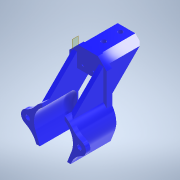
# Autodesk Inventor part: Marco Servo
Saved by Autodesk Inventor 2020.3 (Build 243373000, 373)
## iProperties
Created: 2021-02-18
Part Number: Marco Servo
Material: PET Plastic
Document SubType Name: Modeling
Designer: juanp
Density: 1.541 g/cm^3
Appearance: Polycarbonate - Clear
Author: juanp
Autodesk Inventor part; units mm, degrees
ref_plane "YZ Plane" through (0, 0, 0) normal (1, 0, 0) x (0, 1, 0)
ref_plane "XZ Plane" through (0, 0, 0) normal (0, 1, 0) x (-1, 0, 0)
ref_plane "XY Plane" through (0, 0, 0) normal (0, 0, 1) x (1, 0, 0)
sketch "Sketch1" plane through (0, 0, 0) normal (0, 0, 1) x (1, 0, 0)
  line L0 (0, 0) -> (20, 0)
  line L1 (20, 0) -> (20, 40.2)
  line L2 (20, 40.2) -> (0, 40.2)
  line L3 (0, 40.2) -> (0, 0)
  line L4 (-7, 47.2) -> (27, 47.2)
  line L5 (27, 47.2) -> (27, -7)
  line L6 (27, -7) -> (-7, -7)
  line L7 (-7, -7) -> (-7, 47.2)
  line L8 (10, -7) -> (10, 0) construction
  line L9 (-7, 20.1) -> (0, 20.1) construction
  line L10 (10, 47.2) -> (10, 40.2) construction
  line L11 (20, 20.1) -> (27, 20.1) construction
  line L12 (5.075, -4.611) -> (14.925, -4.611) construction
  line L13 (0.15, 40.05) -> (19.85, 40.05) construction
  line L14 (19.85, 40.05) -> (19.85, 0.15) construction
  line L15 (19.85, 0.15) -> (0.15, 0.15) construction
  line L16 (0.15, 0.15) -> (0.15, 40.05) construction
  line L17 (10, 40.05) -> (10, 40.2) construction
  line L18 (19.85, 20.1) -> (20, 20.1) construction
  line L19 (10, 0.15) -> (10, 0) construction
  line L20 (0, 20.1) -> (0.15, 20.1) construction
  line L21 (5.075, 44.811) -> (14.925, 44.811) construction
  circle A0 centre (5.075, 44.811) radius 0.75
  circle A1 centre (14.925, 44.811) radius 0.75
  circle A2 centre (14.925, -4.611) radius 0.75
  circle A3 centre (5.075, -4.611) radius 0.75
  line L22 (10, 0.15) -> (10, 10) construction
  arc A4 (26.498218, 3.589166) -> (-6.498218, 3.589166) centre (10, 10) ccw
  arc A5 (29.294526, 2.502584) -> (-9.294526, 2.502584) centre (10, 10) ccw
  line L23 (26.498218, 3.589166) -> (22.383508, -7)
  line L24 (-6.498218, 3.589166) -> (-2.383508, -7)
  line L25 (-9.294526, 2.502584) -> (-5.602037, -7)
  line L26 (-5.602037, -7) -> (-2.383508, -7)
  line L27 (22.383508, -7) -> (25.602037, -7)
  line L28 (25.602037, -7) -> (29.294526, 2.502584)
  line L29 (-2.383508, -7) -> (22.383508, -7) construction
  line L30 (10, -7) -> (10, 10) construction
  line L31 (-7, 47.2) -> (-7, 58.9)
  line L32 (-7, 58.9) -> (27, 58.9)
  line L33 (27, 58.9) -> (27, 47.2)
  line L34 (-7, 58.9) -> (27, 58.9)
  line L35 (27, 58.9) -> (27, 54.9)
  line L36 (27, 54.9) -> (-7, 54.9)
  line L37 (-7, 54.9) -> (-7, 58.9)
  line L38 (0, 58.9) -> (0, 54.9)
  line L39 (20, 58.9) -> (20, 54.9)
  line L40 (0, 54.9) -> (0, 47.2)
  line L41 (20, 54.9) -> (20, 47.2)
  point P0 (10, -4.611)
  point P1 (10, 44.811)
  point P2 (-7, 5.071511)
  point P3 (-7, 14.928489)
  point P4 (-7, 21.810588)
  point P5 (27, 21.810588)
  point P6 (27, 14.928489)
  point P7 (27, 5.071511)
  point P8 (0, 28.124293)
  point P9 (0, 24.604451)
  point P10 (20, 28.124293)
  point P11 (20, 24.604451)
  point P12 (-7, -3.402357)
  point P13 (27, -3.402357)
  point P14 (20, 58.9)
  point P15 (0, 58.9)
  dimension "d0" = 40.2
  dimension "d1" = 20
  dimension "d2" = 7
  dimension "d3" = 9.85
  dimension "d4" = 39.9
  dimension "d5" = 4.761
  dimension "d6" = 4.761
  dimension "d7" = 9.85
  dimension "d8" = 1.5
  dimension "d11" = 9.85
  dimension "d12" = 17.7
  dimension "d14" = 3
  dimension "d17" = 42.47
  dimension "d20" = 18.7
  dimension "d21" = 4
  constraints: 84 end point, 16 perpendicular, 15 midpoint, 10 parallel, 10 point on line, 8 horizontal, 6 centre point, 6 coincident, 4 collinear, 4 point on circle, 4 tangent, 3 equal radius, 3 vertical
  measures "d0" distance of L0.end L1.end
  measures "d1" distance of L1.end L2.end
  measures "d2" distance of L10.start L10.end
  measures "d3" distance of L12.start L12.end
  measures "d4" distance of L13.end L14.end
  measures "d5" distance between parallel lines of L15 L12
  measures "d6" distance between parallel lines of L21 L13
  measures "d7" distance of L21.start L21.end
  measures "d8" diameter of A1
  measures "d11" distance of L19.start L22.end
  measures "d12" radius of A4
  measures "d14" radial gap between concentric circles of A5 A4
  measures "d17" angle of L23 L24
  measures "d20" distance between parallel lines of L32 L2
  measures "d21" distance between parallel lines of L32 L36
extrude "Extrusion1" add sketch "Sketch1" along normal blind 5 contours L0 L1 A4 L5 L23 L6 L24 L7 L3 | A4 L7 A5 L3 | L1 A5 L5 A4 | A5 L7 L4 L5 L1 L2 L3 | L7 A4 | A4 L5 | A4 L24 L6 L25 L7 | L5 L28 L6 L23 A4 | L31 L36 L40 L4 | L4 L41 L36 L33 | L40 L36 L41 L4 | L31 L32 L38 L36 | L36 L39 L32 L33 | L38 L32 L39 L36
extrude "Extrusion2" add sketch "Sketch1" along normal blind 36.3 contours A4 L7 A5 L3 | L1 A5 L5 A4 | A4 L7 L25 A5 | L5 A5 L28 A4 | A4 L24 L6 L25 L7 | L5 L28 L6 L23 A4
fillet "Fillet2" radius 5 4 edges at (-4.4409, -1.7054, 5) (-6.91, 15.2288, 5) (24.4409, -1.7054, 5) (26.91, 15.2288, 5)
extrude "Extrusion3" add sketch "Sketch1" against normal blind 30 contours L38 L32 L39 L36
sketch "Sketch3" plane through (20, 54.9, 0) normal (1, 0, 0) x (0, 0, -1)
  line L0 (30, 4) -> (30, 0)
  line L1 (30, 0) -> (0, -30)
  line L2 (0, -14.7) -> (0, -54.9)
  line L3 (0, 0) -> (30, 0)
  line L4 (0, -33.089412) -> (0, 4)
  line L5 (0, 4) -> (30, 4)
  dimension "d24" = 45
  constraints: 2 end point, 1 point on line
  measures "d24" angle of L3 L1
extrude "Extrusion4" add sketch "Sketch3" along normal blind 4
ref_plane "Work Plane1" through (10, 58.9, 0) normal (-1, 0, 0) x (0, 0, 1)
mirror "Mirror1" about plane through (10, 58.9, 0) normal (-1, 0, 0) of "Extrusion4"
chamfer "Chamfer1" distance 3.65 angle 45 5 edges at (20, 54.9, -15) (10, 54.9, 0) (0, 54.9, -15) (0, 12.45, 0) (20, 12.45, 0)
ref_plane "Work Plane3" through (-4, 58.9, 0) normal (-1, 0, 0) x (0, 0, 1)
sketch "Sketch4" plane through (-4, 58.9, 0) normal (-1, 0, 0) x (0, 0, 1)
  line L0 (5, -37.089412) -> (5, 0)
  line L1 (5, -5.789412) -> (36.3, -37.089412)
  line L2 (36.3, -37.089412) -> (5, -37.089412)
  line L3 (36.3, -56.397416) -> (36.3, -30.775707)
  line L4 (5, -30.775707) -> (36.3, -30.775707)
  line L5 (5, -33.652377) -> (36.3, -33.652377)
  line L6 (36.3, -33.652377) -> (36.3, -38.069949)
  line L7 (36.3, -38.069949) -> (10, -38.069949)
  ellipse E0 centre (10, -47.935218) end of major axis (10, -61.739974) minor radius 5 (5.570721, -54.340083) -> (10, -61.739974) ccw
  line L8 (10, -61.739974) -> (36.3, -61.739974)
  line L9 (36.3, -61.739974) -> (36.3, -65.9)
  line L10 (36.3, -65.9) -> (0, -65.9)
  line L11 (0, -65.9) -> (0, -34)
  line L12 (0, -34) -> (0, 0)
  line L13 (-30, 0) -> (0, 0)
  line L14 (-30, -4) -> (-30, 0)
  line L15 (0, -34) -> (-30, -4)
  line L16 (5, 0) -> (5, -33.652377)
  line L17 (0, 0) -> (5, 0)
  point P0 (0, -58.9)
  point P1 (29.986295, -30.775707)
  point P2 (32.862966, -33.652377)
  dimension "d31" = 45
  constraints: 4 end point, 2 point on line, 1 horizontal, 2 other
  measures "d31" angle of L1 L2
extrude "Extrusion5" add sketch "Sketch4" against normal up to surface contours L0 L4 L1 L5 round surface about axis through (10, 10, 0) along (0, 0, 1) radius 20.7 far side no
extrude "Extrusion6" add sketch "Sketch4" against normal up to surface (4 mm away) contours L0 L1 L4
mirror "Mirror2" about plane through (10, 58.9, 0) normal (-1, 0, 0) of "Extrusion6", "Extrusion5"
sketch "Sketch5" plane through (3.65, 54.9, -30) normal (0, -1, 0) x (1, 0, 0)
  line L0 (23.35, 30) -> (20.35, 30) construction
  line L1 (20.35, 30) -> (20.35, 0) construction
  line L2 (20.35, 0) -> (12.7, 0) construction
  line L3 (12.7, 0) -> (12.7, 26.35) construction
  line L4 (12.7, 26.35) -> (0, 26.35) construction
  line L5 (0, 26.35) -> (0, 0) construction
  line L6 (12.7, 0) -> (0, 0) construction
  line L7 (23.35, 35) -> (23.35, 30) construction
  line L8 (-10.65, 35) -> (23.35, 35) construction
  line L9 (-10.65, 30) -> (-10.65, 35) construction
  line L10 (-7.65, 30) -> (-10.65, 30) construction
  line L11 (-7.65, 0) -> (-7.65, 30) construction
  line L12 (0, 0) -> (-7.65, 0) construction
  line L13 (6.35, 26.35) -> (6.35, 20.675) construction
  line L14 (6.35, 20.675) -> (6.35, 5.675) construction
  line L15 (6.35, 5.675) -> (6.35, 0) construction
  circle A0 centre (6.35, 20.675) radius 2.1
  circle A1 centre (6.35, 5.675) radius 2.1
  point P0 (-3.65, 30)
  dimension "d38" = 15
  dimension "d39" = 4.2
  constraints: 6 end point, 2 centre point, 2 coincident, 2 midpoint, 1 collinear, 1 equal radius, 1 point on line, 1 vertical
  measures "d38" distance of L13.end L14.end
  measures "d39" diameter of A0
extrude "Extrusion7" cut sketch "Sketch5" against normal through all
chamfer "Chamfer2" distance 6 angle 45 2 edges at (24, 58.9, -15) (-4, 58.9, -15)
chamfer "Chamfer4" distance 8 angle 45 2 edges at (-7, 58.9, 2.5) (27, 58.9, 2.5)
sketch "Sketch8" plane through (3.65, 54.9, -30) normal (0, -1, 0) x (1, 0, 0)
  line L0 (18.35, 0) -> (12.7, 0) projected
  line L1 (12.7, 0) -> (0, 0) projected
  line L2 (0, 0) -> (-5.65, 0) projected
  line L3 (-5.65, 0) -> (-5.65, 30) projected
  line L4 (-5.65, 30) -> (-6.65, 30) projected
  line L5 (-6.65, 30) -> (-6.65, 35) projected
  line L6 (-6.65, 35) -> (19.35, 35) projected
  line L7 (19.35, 35) -> (19.35, 30) projected
  line L8 (19.35, 30) -> (18.35, 30) projected
  line L9 (18.35, 30) -> (18.35, 0) projected
  line L10 (12.7, 0) -> (12.7, 26.35) projected
  line L11 (12.7, 26.35) -> (0, 26.35) projected
  line L12 (0, 26.35) -> (0, 0) projected
  circle A0 centre (6.35, 20.675) radius 2.1 projected
  circle A1 centre (6.35, 5.675) radius 2.1 projected
  line L13 (12.7, 18.575) -> (0, 18.575)
  line L14 (12.7, 22.775) -> (0, 22.775)
  line L15 (12.7, 7.775) -> (0, 7.775)
  line L16 (12.7, 3.575) -> (0, 3.575)
  line L17 (4.25, 7.775) -> (8.45, 7.775)
  line L18 (8.45, 7.775) -> (8.45, 3.575)
  line L19 (8.45, 3.575) -> (4.25, 3.575)
  line L20 (4.25, 3.575) -> (4.25, 7.775)
  line L21 (4.25, 7.775) -> (8.45, 3.575) construction
  line L22 (8.45, 7.775) -> (4.25, 3.575) construction
  line L23 (4.25, 22.775) -> (8.45, 22.775)
  line L24 (8.45, 22.775) -> (8.45, 18.575)
  line L25 (8.45, 18.575) -> (4.25, 18.575)
  line L26 (4.25, 18.575) -> (4.25, 22.775)
  line L27 (4.25, 22.775) -> (8.45, 18.575) construction
  line L28 (8.45, 22.775) -> (4.25, 18.575) construction
  circle A2 centre (6.35, 5.675) radius 2.1 projected
  circle A3 centre (6.35, 20.675) radius 2.1 projected
  point P0 (-3.65, 30)
  point P1 (4.25, 22.775)
  point P2 (4.25, 18.575)
  point P3 (4.25, 7.775)
  point P4 (4.25, 3.575)
  point P5 (4.25, 20.675)
  point P6 (6.35, 18.575)
  point P7 (6.35, 22.775)
  point P8 (8.45, 20.675)
  point P9 (4.25, 5.675)
  point P10 (6.35, 3.575)
  point P11 (6.35, 7.775)
  point P12 (8.45, 5.675)
  constraints: 32 end point, 10 point on line, 6 tangent, 5 parallel, 5 perpendicular, 4 midpoint, 2 horizontal
extrude "Extrusion10" cut sketch "Sketch8" against normal blind 0.3 contours L16 L18 L15 L10 | L12 L15 L20 L16 | L13 L24 L14 L10 | L12 L14 L26 L13
extrude "Extrusion11" cut sketch "Sketch8" against normal blind 0.6 contours L16 A1 L18 | L20 A1 L16 | L18 A1 L15 | L15 A1 L20 | L13 A0 L24 | L26 A0 L13 | L24 A0 L14 | L14 A0 L26
sketch "Sketch9" plane through (0, 0, 36.3) normal (0, 0, 1) x (1, 0, 0)
  arc A0 (29.294526, 2.502584) -> (20, 28.124293) centre (10, 10) ccw
  line L0 (10, 10) -> (33.5, 10) construction
  circle A1 centre (33.5, 10) radius 2
  arc A2 (29.294526, 2.502584) -> (27, 21.810588) centre (10, 10) ccw
  line L1 (29.81136, 4) -> (33.5, 4)
  line L2 (29.81136, 16) -> (33.5, 16)
  arc A3 (33.5, 4) -> (33.5, 16) centre (33.5, 10) ccw
  line L3 (10, 10) -> (10, 16)
  arc A4 (0, 28.124293) -> (-9.294526, 2.502584) centre (10, 10) ccw
  circle A5 centre (-13.5, 10) radius 2
  line L4 (-9.81136, 4) -> (-13.5, 4)
  line L5 (-9.81136, 16) -> (-13.5, 16)
  arc A6 (-13.5, 16) -> (-13.5, 4) centre (-13.5, 10) ccw
  point P0 (0, 0)
  dimension "d63" = 23.5
  dimension "d64" = 4
  dimension "d65" = 4
  constraints: 12 end point, 7 symmetric about line, 6 point on circle, 4 centre point, 3 horizontal, 2 coincident, 2 tangent, 1 concentric, 1 parallel, 1 vertical, 2 other
  measures "d63" distance of L0.start L0.end
  measures "d64" diameter of A1
  measures "d65" radial gap between concentric circles of A3 A1
extrude "Extrusion12" add sketch "Sketch9" against normal blind 4
fillet "Fillet5" radius 20 4 edges at (-9.8114, 4, 34.3) (29.8114, 4, 34.3) (-9.8114, 16, 34.3) (29.8114, 16, 34.3)
sketch "Sketch10" plane through (0, 0, 32.3) normal (0, 0, -1) x (-1, 0, 0)
  circle A0 centre (-33.5, 10) radius 2
  circle A1 centre (13.5, 10) radius 2
  circle A2 centre (-33.5, 10) radius 2
  line L0 (-35.506292, 13.475) -> (-31.493708, 13.475)
  line L1 (-31.493708, 13.475) -> (-29.487416, 10)
  line L2 (-29.487416, 10) -> (-31.493708, 6.525)
  line L3 (-31.493708, 6.525) -> (-35.506292, 6.525)
  line L4 (-35.506292, 6.525) -> (-37.512584, 10)
  line L5 (-37.512584, 10) -> (-35.506292, 13.475)
  line L6 (11.493708, 6.525) -> (9.487416, 10)
  line L7 (9.487416, 10) -> (11.493708, 13.475)
  line L8 (11.493708, 13.475) -> (15.506292, 13.475)
  line L9 (15.506292, 13.475) -> (17.512584, 10)
  line L10 (17.512584, 10) -> (15.506292, 6.525)
  line L11 (15.506292, 6.525) -> (11.493708, 6.525)
  point P0 (0, 0)
  dimension "d69" = 6.95
  constraints: 24 end point, 2 coincident, 2 collinear, 26 other
  measures "d69" distance between parallel lines of L8 L11
extrude "Extrusion13" cut sketch "Sketch10" along normal blind 4 and the other way blind 2
body "Solid1"
